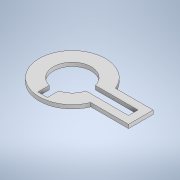
# Autodesk Inventor part: Pièce_maintient_test_4.1
Saved by Autodesk Inventor 2020.1 (Build 241239000, 239)
## iProperties
Created: 2019-08-18
Part Number: Pièce_maintient_test_4.1
Material: Générique
Document SubType Name: Modeling
Designer: marlo
Density: 1 g/cm^3
Appearance: Par défaut
Author: marlo
Autodesk Inventor part; units mm, degrees
ref_plane "YZ Plane" through (0, 0, 0) normal (1, 0, 0) x (0, 1, 0)
ref_plane "XZ Plane" through (0, 0, 0) normal (0, 1, 0) x (-1, 0, 0)
ref_plane "XY Plane" through (0, 0, 0) normal (0, 0, 1) x (1, 0, 0)
sketch "Esquisse1" plane through (0, 0, 0) normal (0, 1, 0) x (-1, 0, 0)
  circle A0 centre (0, 0) radius 10
  circle A1 centre (0, 0) radius 17.5
  line L0 (2.5, 15.6825) -> (-2.5, 15.6825)
  line L1 (-2.5, 15.6825) -> (-2.5, 9.6825)
  line L2 (-2.5, 9.6825) -> (2.5, 9.6825)
  line L3 (2.5, 9.6825) -> (2.5, 15.6825)
  line L4 (-32.1825, 2.5) -> (-9.6825, 2.5)
  line L5 (-9.6825, 2.5) -> (-9.6825, -2.5)
  line L6 (-9.6825, -2.5) -> (-32.1825, -2.5)
  line L7 (-32.1825, -2.5) -> (-32.1825, 2.5)
  line L8 (-36.1825, -6.5) -> (-5.6825, -6.5)
  line L9 (-5.6825, -6.5) -> (-5.6825, 6.5)
  line L10 (-5.6825, 6.5) -> (-36.1825, 6.5)
  line L11 (-36.1825, 6.5) -> (-36.1825, -6.5)
  point P0 (-16.2481, -6.5)
  point P1 (-16.2481, 6.5)
  dimension "d0" = 20
  dimension "d1" = 35
  dimension "d2" = 5
  dimension "d3" = 6
  dimension "d4" = 5
  dimension "d5" = 22.5
  dimension "d6" = 4
  constraints: 24 end point, 6 parallel, 4 point on circle, 3 perpendicular, 2 centre point, 2 horizontal, 1 coincident, 3 other
  measures "d0" diameter of A0
  measures "d1" diameter of A1
  measures "d2" distance of L0.start L0.end
  measures "d3" distance of L2.end L0.start
  measures "d4" distance of L6.end L4.start
  measures "d5" distance of L5.end L6.end
  measures "d6" distance between parallel lines of L6 L8
extrude "Extrusion1" add sketch "Esquisse1" along normal blind 2 contours A0 L3 L0 L1 L10 A1 L8 | L8 A1 L6 A0 | L8 L11 L10 A1 L4 L7 L6 | A0 L4 A1 L10
